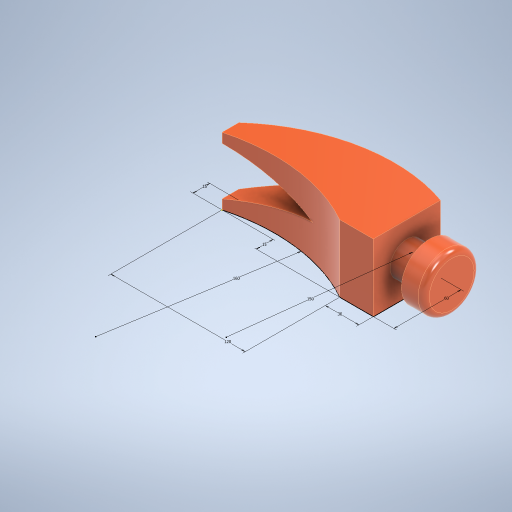
# Autodesk Inventor part: practice3
Saved by Autodesk Inventor 2024 (Build 280153000, 153)
## iProperties
Created: 2024-02-14
Part Number: practice3
Material: Phenolharz
Document SubType Name: Modeling
Designer: ffogue
Density: 1.38 g/cm^3
Appearance: Glatt - Hellorange
Mass: 588.87 g
Surface Area: 460.242 cm^2
Volume: 426.718 cm^3
BeforeDocSave0: Durchmesser
Author: ffogue
Autodesk Inventor part; units mm, degrees
ref_plane "YZ Plane" through (0, 0, 0) normal (1, 0, 0) x (0, 1, 0)
ref_plane "XZ Plane" through (0, 0, 0) normal (0, 1, 0) x (-1, 0, 0)
sketch "Skizze1" plane through (0, 0, 0) normal (0, 0, 1) x (1, 0, 0)
  line L0 (0, 0) -> (0, 15)
  arc A0 (150, 45) -> (0, 15) centre (100.3058, -96.5291) ccw
  line L1 (150, 45) -> (150, -15)
  line L2 (150, -15) -> (120, -15)
  arc A1 (120, -15) -> (0, 0) centre (41.6262, -154.4903) ccw
  dimension "hoehe2" = 60
  dimension "Durchmesser" = 160
  dimension "Durchmesser2" = 150
  dimension "Breite1" = 30
  dimension "d12" = 120
  dimension "Höhe1" = 15
  dimension "d14" = 15
  constraints: 6 end point, 4 point on circle, 2 centre point, 2 vertical, 1 coincident, 1 perpendicular
  measures "hoehe2" distance of L1.start L1.end
  measures "Durchmesser" radius of A1
  measures "Durchmesser2" radius of A0
  measures "Breite1" distance of L1.end L2.end
  measures "d12" horizontal distance of L2.end L0.start
  measures "Höhe1" distance of L0.start L0.end
  measures "d14" distance from line of L2 L0.start
extrude "Extrusion1" add sketch "Skizze1" along normal blind 60
ref_plane "Arbeitsebene1" through (100.3058, 53.4709, 0) normal (0, -1, 0) x (1, 0, 0)
sketch "Skizze2" plane through (100.3058, 53.4709, 0) normal (0, -1, 0) x (1, 0, 0)
  line L0 (-100.3058, 0) -> (-100.3058, 60) projected
  line L1 (-100.3058, 51.4359) -> (-20.3058, 30)
  line L2 (-20.3058, 30) -> (-100.3058, 8.5641)
  line L3 (-100.3058, 30) -> (-9.7877, 30) construction
  dimension "d17" = 30
  dimension "d18" = 80
  constraints: 6 end point, 3 point on line, 1 horizontal, 1 midpoint, 1 symmetric about line
  measures "d17" angle of L2 L1
  measures "d18" distance from line of L0 L1.end
extrude "Extrusion2" cut sketch "Skizze2" along normal up to surface
sketch "Skizze3" plane through (150, -15, 0) normal (1, 0, 0) x (0, 0, -1)
  circle A0 centre (-30, 30) radius 15
  line L0 (0, 0) -> (0, 60) projected
  line L1 (0, 0) -> (-60, 0) projected
  point P0 (0, 15)
  point P1 (0, 30)
  point P2 (-30, 0)
  dimension "d21" = 30
  constraints: 2 midpoint, 1 centre point, 1 horizontal alignment, 1 vertical alignment
  measures "d21" diameter of A0
extrude "Extrusion3" add sketch "Skizze3" along normal blind 20
sketch "Skizze4" plane through (170, 15, 30) normal (1, 0, 0) x (0, 0, -1)
  line L0 (0, 37.0901) -> (0, -14.1602) projected
  circle A0 centre (0, 0) radius 25
  line L1 (30, -30) -> (30, 30) projected
  point P0 (30, -15)
  point P1 (30, 0)
  dimension "d24" = 50
  constraints: 1 centre point, 1 horizontal alignment, 1 midpoint, 1 point on line
  measures "d24" diameter of A0
extrude "Extrusion4" add sketch "Skizze4" along normal blind 20
fillet "Rundung1" radius 5 1 edges at (190, 15, 55)
